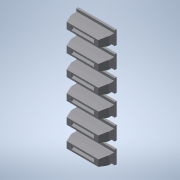
# Autodesk Inventor part: 0088-02-r2-coin-buttons-panelmot
Saved by Autodesk Inventor 2020.2 (Build 242310000, 310)
## iProperties
Created: 2011-08-20
Part Number: 0088-02-r2-coin-buttons-panelmot
Material: Allgemein
Document SubType Name: Modeling
Designer: Jaso
Density: 1 g/cm^3
Appearance: Vorgabe
Author: Jaso
Autodesk Inventor part; units mm, degrees
ref_plane "YZ Plane" through (0, 0, 0) normal (1, 0, 0) x (0, 1, 0)
ref_plane "XZ Plane" through (0, 0, 0) normal (0, 1, 0) x (-1, 0, 0)
sketch "Sketch1" plane through (0, 0, 0) normal (0, 0, 1) x (1, 0, 0)
  line L0 (-18.796, 63.5) -> (18.796, 63.5)
  line L1 (18.796, 63.5) -> (18.796, -63.5)
  line L2 (18.796, -63.5) -> (-18.796, -63.5)
  line L3 (-18.796, -63.5) -> (-18.796, 63.5)
  point P0 (0, 0)
  point P1 (18.796, 0)
  point P2 (0, 63.5)
  dimension "d0" = 127
  dimension "d1" = 37.592
  constraints: 8 end point, 2 midpoint, 2 parallel, 1 horizontal, 1 horizontal alignment, 1 perpendicular, 1 vertical alignment
  measures "d0" distance of L0.end L1.end
  measures "d1" distance between parallel lines of L3 L1
extrude "Extrusion1" add sketch "Sketch1" along normal blind 3.175
sketch "Sketch5" plane through (0, 0, 3.175) normal (0, 0, 1) x (1, 0, 0)
  line L0 (18.796, -63.5) -> (-18.796, -63.5) projected
  point P0 (0, 0)
  point P1 (0, -59.5376)
  point P2 (0, 59.5376)
  dimension "d22" = 119.0752
  dimension "d23" = 3.9624
  constraints: 2 vertical alignment
  measures "d22" distance of point (0, 59.538) point (0, -59.538)
  measures "d23" distance from line of point (0, -59.538) L0
hole "Hole1" at (0, -59.5376, 3.175) at (0, 59.5376, 3.175) direction (0, 0, -1) diameter 3.175 end through all
sketch "Sketch2" plane through (0, 0, 3.175) normal (0, 0, 1) x (1, 0, 0)
  line L0 (18.796, 63.5) -> (18.796, -63.5) projected
  line L1 (-18.796, -63.5) -> (-18.796, 63.5) projected
  line L2 (18.796, -63.5) -> (-18.796, -63.5) projected
  line L3 (-18.796, -45.8978) -> (18.796, -45.8978)
  line L4 (18.796, -45.8978) -> (18.796, -55.0418)
  line L5 (18.796, -55.0418) -> (-18.796, -55.0418)
  line L6 (-18.796, -55.0418) -> (-18.796, -45.8978)
  point P0 (0, 0)
  dimension "d4" = 9.144
  dimension "d5" = 8.4582
  constraints: 8 end point, 2 parallel, 2 point on line, 1 horizontal, 1 perpendicular
  measures "d4" distance between parallel lines of L3 L5
  measures "d5" distance between parallel lines of L5 L2
extrude "Extrusion2" add sketch "Sketch2" along normal blind 12.7 contours L0 L5 L1 L3
ref_plane "Work Plane1" through (0, 0, 24.8412) normal (0, 0, 1) x (1, 0, 0)
sketch "Sketch3" plane through (0, 0, 24.8412) normal (0, 0, 1) x (1, 0, 0)
  line L0 (18.796, -55.0418) -> (-18.796, -55.0418) projected
  line L1 (18.796, -45.8978) -> (18.796, -55.0418) projected
  line L2 (-18.796, -45.8978) -> (18.796, -45.8978) projected
  line L3 (-18.796, -55.0418) -> (-18.796, -45.8978) projected
  line L4 (-15.5321, -47.2948) -> (15.5321, -47.2948)
  line L5 (15.5321, -47.2948) -> (15.5321, -53.6448)
  line L6 (15.5321, -53.6448) -> (-15.5321, -53.6448)
  line L7 (-15.5321, -53.6448) -> (-15.5321, -47.2948)
  point P0 (0, 0)
  point P1 (15.5321, -50.4698)
  point P2 (18.796, -50.4698)
  point P3 (0, -45.8978)
  point P4 (0, -47.2948)
  dimension "d9" = 31.0642
  dimension "d10" = 6.35
  constraints: 8 end point, 4 midpoint, 2 parallel, 1 horizontal, 1 horizontal alignment, 1 perpendicular, 1 vertical alignment
  measures "d9" distance of L4.start L4.end
  measures "d10" distance of L4.end L5.end
loft "Loft1" add profiles "Sketch3" section 2 edges at (0, -55.0418, 15.875) (18.796, -50.4698, 15.875) (0, -45.8978, 15.875) (-18.796, -50.4698, 15.875) contours L4 L5 L6 L7
sketch "Sketch4" plane through (-15.5321, -47.2948, 24.8412) normal (0, 0, 1) x (1, 0, 0)
  line L0 (0, 0) -> (31.0642, 0) projected
  line L1 (31.0642, 0) -> (31.0642, -6.35) projected
  line L2 (4.4196, -1.5875) -> (26.6446, -1.5875)
  line L3 (26.6446, -1.5875) -> (26.6446, -4.7625)
  line L4 (26.6446, -4.7625) -> (4.4196, -4.7625)
  line L5 (4.4196, -4.7625) -> (4.4196, -1.5875)
  point P0 (15.5321, 47.2948)
  point P1 (26.6446, -3.175)
  point P2 (31.0642, -3.175)
  point P3 (15.5321, -1.5875)
  point P4 (15.5321, 0)
  dimension "d15" = 3.175
  dimension "d16" = 22.225
  constraints: 8 end point, 4 midpoint, 2 parallel, 1 horizontal, 1 horizontal alignment, 1 perpendicular, 1 vertical alignment
  measures "d15" distance of L2.end L3.end
  measures "d16" distance of L2.start L2.end
extrude "Extrusion3" cut sketch "Sketch4" against normal through all
pattern_linear "Rectangular Pattern1" count 6 spacing 20.193 along (0, 1, 0) of "Extrusion2", "Loft1", "Extrusion3"
sketch "Skizze6" plane through (0, 0, 3.175) normal (0, 0, 1) x (1, 0, 0)
  line L0 (-24.1756, 43.8912) -> (26.7048, 43.8912)
  line L1 (26.7048, 43.8912) -> (26.7048, 36.9062)
  line L2 (26.7048, 36.9062) -> (-24.1756, 36.9062)
  line L3 (-24.1756, 36.9062) -> (-24.1756, 43.8912)
  line L4 (-24.1756, 23.6982) -> (26.7048, 23.6982)
  line L5 (26.7048, 23.6982) -> (26.7048, 16.7132)
  line L6 (26.7048, 16.7132) -> (-24.1756, 16.7132)
  line L7 (-24.1756, 16.7132) -> (-24.1756, 23.6982)
  line L8 (-24.1756, 3.5052) -> (26.7048, 3.5052)
  line L9 (26.7048, 3.5052) -> (26.7048, -3.4798)
  line L10 (26.7048, -3.4798) -> (-24.1756, -3.4798)
  line L11 (-24.1756, -3.4798) -> (-24.1756, 3.5052)
  line L12 (-24.1756, -16.6878) -> (26.7048, -16.6878)
  line L13 (26.7048, -16.6878) -> (26.7048, -23.6728)
  line L14 (26.7048, -23.6728) -> (-24.1756, -23.6728)
  line L15 (-24.1756, -23.6728) -> (-24.1756, -16.6878)
  line L16 (-24.1756, 57.0992) -> (26.7048, 57.0992)
  line L17 (26.7048, 57.0992) -> (26.7048, 65.0866)
  line L18 (26.7048, 65.0866) -> (-24.1756, 65.0866)
  line L19 (-24.1756, 65.0866) -> (-24.1756, 57.0992)
  line L20 (-24.1756, -36.8808) -> (26.7048, -36.8808)
  line L21 (26.7048, -36.8808) -> (26.7048, -43.8658)
  line L22 (26.7048, -43.8658) -> (-24.1756, -43.8658)
  line L23 (-24.1756, -43.8658) -> (-24.1756, -36.8808)
  line L24 (-24.1756, -57.0738) -> (26.7048, -57.0738)
  line L25 (26.7048, -57.0738) -> (26.7048, -65.8307)
  line L26 (26.7048, -65.8307) -> (-24.1756, -65.8307)
  line L27 (-24.1756, -65.8307) -> (-24.1756, -57.0738)
  line L28 (-18.796, 55.0672) -> (18.796, 55.0672) projected
  line L29 (18.796, 45.9232) -> (-18.796, 45.9232) projected
  line L30 (-18.796, 34.8742) -> (18.796, 34.8742) projected
  line L31 (18.796, 25.7302) -> (-18.796, 25.7302) projected
  line L32 (-18.796, 14.6812) -> (18.796, 14.6812) projected
  line L33 (18.796, 5.5372) -> (-18.796, 5.5372) projected
  line L34 (-18.796, -5.5118) -> (18.796, -5.5118) projected
  line L35 (18.796, -14.6558) -> (-18.796, -14.6558) projected
  line L36 (-18.796, -25.7048) -> (18.796, -25.7048) projected
  line L37 (18.796, -34.8488) -> (-18.796, -34.8488) projected
  line L38 (-18.796, -45.8978) -> (18.796, -45.8978) projected
  line L39 (18.796, -55.0418) -> (-18.796, -55.0418) projected
  point P0 (0, 0)
  dimension "d31" = 2.032
  dimension "d32" = 2.032
  dimension "d33" = 2.032
  dimension "d34" = 2.032
  dimension "d35" = 2.032
  dimension "d36" = 2.032
  dimension "d37" = 2.032
  dimension "d38" = 2.032
  dimension "d39" = 2.032
  dimension "d40" = 2.032
  dimension "d41" = 2.032
  dimension "d42" = 2.032
  constraints: 56 end point, 14 parallel, 11 point on line, 7 horizontal, 7 perpendicular
  measures "d31" distance between parallel lines of L16 L28
  measures "d32" distance between parallel lines of L29 L0
  measures "d33" distance between parallel lines of L30 L2
  measures "d34" distance between parallel lines of L31 L4
  measures "d35" distance between parallel lines of L6 L32
  measures "d36" distance between parallel lines of L8 L33
  measures "d37" distance between parallel lines of L34 L10
  measures "d38" distance between parallel lines of L35 L12
  measures "d39" distance between parallel lines of L36 L14
  measures "d40" distance from line of L37 L20.end
  measures "d41" distance between parallel lines of L22 L38
  measures "d42" distance between parallel lines of L24 L39
extrude "Extrusion4" cut sketch "Skizze6" against normal blind 25.4
sketch "Skizze7" plane through (0, 0, 0) normal (0, 0, -1) x (-1, 0, 0)
  line L0 (18.796, 57.0992) -> (-18.796, 57.0992) projected
  line L1 (-18.796, 57.0992) -> (-18.796, 43.8912) projected
  line L2 (-18.796, 43.8912) -> (18.796, 43.8912) projected
  line L3 (18.796, 43.8912) -> (18.796, 57.0992) projected
  line L4 (-18.796, 55.0672) -> (-18.796, 45.9232) projected
  line L5 (-18.796, 50.4952) -> (18.796, 50.4952) construction
  line L6 (-11.1125, 48.9077) -> (-11.1125, 52.0827) projected
  circle A0 centre (-11.1125, 50.4952) radius 2
  line L7 (11.1125, 52.0827) -> (11.1125, 48.9077) projected
  circle A1 centre (11.1125, 50.4952) radius 2
  point P0 (0, 0)
  dimension "d45" = 4
  dimension "d46" = 4
  constraints: 4 midpoint, 2 centre point, 2 end point
  measures "d45" diameter of A0
  measures "d46" diameter of A1
extrude "Extrusion5" cut sketch "Skizze7" against normal blind 22.86 contours A0 | A1
sketch "Skizze8" plane through (0, 0, 0) normal (0, 0, -1) x (-1, 0, 0)
  line L0 (-1.9907, 52.4486) -> (2.0093, 52.4486)
  line L1 (2.0093, 52.4486) -> (2.0093, 48.4486)
  line L2 (2.0093, 48.4486) -> (-1.9907, 48.4486)
  line L3 (-1.9907, 48.4486) -> (-1.9907, 52.4486)
  line L4 (-1.9907, 52.4486) -> (2.0093, 48.4486) construction
  line L5 (2.0093, 52.4486) -> (-1.9907, 48.4486) construction
  point P0 (0, 0)
  point P1 (0.0093, 50.4486)
  dimension "d49" = 4
  dimension "d50" = 4
  constraints: 12 end point, 2 midpoint, 2 parallel, 1 horizontal, 1 perpendicular
  measures "d49" distance of L1.end L2.end
  measures "d50" distance of L0.end L1.end
extrude "Extrusion6" add sketch "Skizze8" against normal blind 5
sketch "Skizze10" plane through (0, 0, 0) normal (0, 0, -1) x (-1, 0, 0)
  line L0 (-19.2035, 30.2914) -> (18.796, 30.3022) construction
  line L1 (18.796, 23.6982) -> (18.796, 36.9062) projected
  line L2 (-19.1977, 9.8718) -> (18.796, 9.8718) construction
  line L3 (-18.796, -3.4798) -> (-18.796, -16.6878) projected
  line L4 (-18.796, -10.0838) -> (18.796, -10.0838) construction
  line L5 (-18.796, -23.6728) -> (-18.796, -36.8808) projected
  line L6 (-18.796, -30.2768) -> (18.796, -30.2768) construction
  line L7 (-18.796, -45.8978) -> (-18.796, -55.0418) projected
  line L8 (-18.796, -50.4698) -> (18.796, -50.4698) construction
  circle A0 centre (-11.0557, 30.2937) radius 2
  line L9 (11.1125, 31.8897) -> (11.1125, 28.7147) construction
  circle A1 centre (11.1125, 30.3022) radius 2
  line L10 (-11.1125, 8.5217) -> (-11.1125, 11.6967) construction
  circle A2 centre (-11.1125, 10.1092) radius 2
  line L11 (11.1125, 8.5217) -> (11.1125, 11.6967) construction
  circle A3 centre (11.1125, 10.1092) radius 2
  line L12 (-11.1125, -8.4963) -> (-11.1125, -11.6713) projected
  circle A4 centre (-11.1125, -10.0838) radius 2
  circle A5 centre (11.1125, -10.0838) radius 2
  line L13 (-11.1125, -31.8643) -> (-11.1125, -28.6893) projected
  circle A6 centre (-11.1125, -30.2768) radius 2
  line L14 (11.1125, -28.6893) -> (11.1125, -31.8643) projected
  circle A7 centre (11.1125, -30.2768) radius 2
  line L15 (-11.1125, -52.0573) -> (-11.1125, -48.8823) projected
  circle A8 centre (-11.1125, -50.4698) radius 2
  line L16 (11.1125, -48.8823) -> (11.1125, -52.0573) projected
  circle A9 centre (11.1125, -50.4698) radius 2
  point P0 (0, 0)
  dimension "d53" = 4
  dimension "d54" = 4
  dimension "d55" = 4
  dimension "d56" = 4
  dimension "d57" = 4
  dimension "d58" = 4
  dimension "d59" = 4
  dimension "d60" = 4
  dimension "d61" = 4
  dimension "d62" = 4
  constraints: 12 midpoint, 10 centre point, 10 end point, 4 horizontal, 2 point on line
  measures "d53" diameter of A0
  measures "d54" diameter of A1
  measures "d55" diameter of A2
  measures "d56" diameter of A3
  measures "d57" diameter of A4
  measures "d58" diameter of A5
  measures "d59" diameter of A6
  measures "d60" diameter of A7
  measures "d61" diameter of A8
  measures "d62" diameter of A9
extrude "Extrusion7" cut sketch "Skizze10" against normal blind 22.86
sketch "Skizze11" plane through (0, 0, 0) normal (0, 0, -1) x (-1, 0, 0)
  line L0 (-1.9772, 32.2984) -> (2.0228, 32.2984)
  line L1 (2.0228, 32.2984) -> (2.0228, 28.2984)
  line L2 (2.0228, 28.2984) -> (-1.9772, 28.2984)
  line L3 (-1.9772, 28.2984) -> (-1.9772, 32.2984)
  line L4 (-1.9772, 32.2984) -> (2.0228, 28.2984) construction
  line L5 (2.0228, 32.2984) -> (-1.9772, 28.2984) construction
  line L6 (-1.9661, 12.2651) -> (2.0339, 12.2651)
  line L7 (2.0339, 12.2651) -> (2.0339, 8.0041)
  line L8 (2.0339, 8.0041) -> (-1.9661, 8.0041)
  line L9 (-1.9661, 8.0041) -> (-1.9661, 12.2651)
  line L10 (-1.9661, 12.2651) -> (2.0339, 8.0041) construction
  line L11 (2.0339, 12.2651) -> (-1.9661, 8.0041) construction
  line L12 (-1.9772, -8.2024) -> (2.0228, -8.2024)
  line L13 (2.0228, -8.2024) -> (2.0228, -12.2024)
  line L14 (2.0228, -12.2024) -> (-1.9772, -12.2024)
  line L15 (-1.9772, -12.2024) -> (-1.9772, -8.2024)
  line L16 (-1.9772, -8.2024) -> (2.0228, -12.2024) construction
  line L17 (2.0228, -8.2024) -> (-1.9772, -12.2024) construction
  line L18 (-1.9772, -27.9157) -> (2.0228, -27.9157)
  line L19 (2.0228, -27.9157) -> (2.0228, -31.9157)
  line L20 (2.0228, -31.9157) -> (-1.9772, -31.9157)
  line L21 (-1.9772, -31.9157) -> (-1.9772, -27.9157)
  line L22 (-1.9772, -27.9157) -> (2.0228, -31.9157) construction
  line L23 (2.0228, -27.9157) -> (-1.9772, -31.9157) construction
  line L24 (-1.9772, -48.7043) -> (2.0228, -48.7043)
  line L25 (2.0228, -48.7043) -> (2.0228, -52.7043)
  line L26 (2.0228, -52.7043) -> (-1.9772, -52.7043)
  line L27 (-1.9772, -52.7043) -> (-1.9772, -48.7043)
  line L28 (-1.9772, -48.7043) -> (2.0228, -52.7043) construction
  line L29 (2.0228, -48.7043) -> (-1.9772, -52.7043) construction
  point P0 (0, 0)
  point P1 (0.0228, 30.2984)
  point P2 (0.0339, 10.1346)
  point P3 (0.0228, -10.2024)
  point P4 (0.0228, -29.9157)
  point P5 (0.0228, -50.7043)
  dimension "d65" = 4
  dimension "d66" = 4
  dimension "d67" = 4
  dimension "d68" = 4
  dimension "d69" = 4
  dimension "d70" = 4
  dimension "d71" = 4
  dimension "d72" = 4
  dimension "d73" = 4
  constraints: 60 end point, 10 midpoint, 10 parallel, 5 horizontal, 5 perpendicular
  measures "d65" distance of L1.end L2.end
  measures "d66" distance of L0.end L1.end
  measures "d67" distance of L7.end L8.end
  measures "d68" distance of L13.end L14.end
  measures "d69" distance of L12.end L13.end
  measures "d70" distance of L19.end L20.end
  measures "d71" distance of L18.end L19.end
  measures "d72" distance of L25.end L26.end
  measures "d73" distance of L24.end L25.end
extrude "Extrusion8" add sketch "Skizze11" against normal blind 5
sketch "Skizze12" plane through (-15.5321, 53.6702, 24.8412) normal (0, 0, 1) x (1, 0, 0)
  line L0 (-3.2639, 1.397) -> (34.3281, 1.397) projected
  line L1 (-3.2639, -7.747) -> (-3.2639, 1.397) projected
  line L2 (34.3281, -7.747) -> (-3.2639, -7.747) projected
  line L3 (34.3281, 1.397) -> (34.3281, -7.747) projected
  line L4 (-3.2639, -18.796) -> (34.3281, -18.796) projected
  line L5 (34.3281, -18.796) -> (34.3281, -27.94) projected
  line L6 (34.3281, -27.94) -> (-3.2639, -27.94) projected
  line L7 (-3.2639, -27.94) -> (-3.2639, -18.796) projected
  line L8 (-3.2639, -38.989) -> (34.3281, -38.989) projected
  line L9 (34.3281, -38.989) -> (34.3281, -48.133) projected
  line L10 (34.3281, -48.133) -> (-3.2639, -48.133) projected
  line L11 (-3.2639, -48.133) -> (-3.2639, -38.989) projected
  line L12 (-3.2639, -59.182) -> (34.3281, -59.182) projected
  line L13 (34.3281, -59.182) -> (34.3281, -68.326) projected
  line L14 (34.3281, -68.326) -> (-3.2639, -68.326) projected
  line L15 (-3.2639, -68.326) -> (-3.2639, -59.182) projected
  line L16 (-3.2639, -79.375) -> (34.3281, -79.375) projected
  line L17 (34.3281, -79.375) -> (34.3281, -88.519) projected
  line L18 (34.3281, -88.519) -> (-3.2639, -88.519) projected
  line L19 (-3.2639, -88.519) -> (-3.2639, -79.375) projected
  line L20 (-3.2639, -99.568) -> (34.3281, -99.568) projected
  line L21 (-3.2639, -108.712) -> (-3.2639, -99.568) projected
  line L22 (34.3281, -108.712) -> (-3.2639, -108.712) projected
  line L23 (34.3281, -99.568) -> (34.3281, -108.712) projected
  line L24 (33.8281, 0.897) -> (-2.7639, 0.897)
  line L25 (-2.7639, 0.897) -> (-2.7639, -7.247)
  line L26 (-2.7639, -7.247) -> (33.8281, -7.247)
  line L27 (33.8281, -7.247) -> (33.8281, 0.897)
  line L28 (33.8281, -19.296) -> (-2.7639, -19.296)
  line L29 (-2.7639, -19.296) -> (-2.7639, -27.44)
  line L30 (-2.7639, -27.44) -> (33.8281, -27.44)
  line L31 (33.8281, -27.44) -> (33.8281, -19.296)
  line L32 (33.8281, -39.489) -> (-2.7639, -39.489)
  line L33 (-2.7639, -39.489) -> (-2.7639, -47.633)
  line L34 (-2.7639, -47.633) -> (33.8281, -47.633)
  line L35 (33.8281, -47.633) -> (33.8281, -39.489)
  line L36 (33.8281, -59.682) -> (-2.7639, -59.682)
  line L37 (-2.7639, -59.682) -> (-2.7639, -67.826)
  line L38 (-2.7639, -67.826) -> (33.8281, -67.826)
  line L39 (33.8281, -67.826) -> (33.8281, -59.682)
  line L40 (33.8281, -79.875) -> (-2.7639, -79.875)
  line L41 (-2.7639, -79.875) -> (-2.7639, -88.019)
  line L42 (-2.7639, -88.019) -> (33.8281, -88.019)
  line L43 (33.8281, -88.019) -> (33.8281, -79.875)
  line L44 (33.8281, -100.068) -> (-2.7639, -100.068)
  line L45 (-2.7639, -100.068) -> (-2.7639, -108.212)
  line L46 (-2.7639, -108.212) -> (33.8281, -108.212)
  line L47 (33.8281, -108.212) -> (33.8281, -100.068)
  point P0 (15.5321, -53.6702)
  dimension "d76" = 0.5
  dimension "d77" = 0.5
  dimension "d78" = 0.5
  dimension "d79" = 0.5
  dimension "d80" = 0.5
  dimension "d81" = 0.5
  constraints: 48 end point, 18 other
  measures "d76" distance between parallel lines of L0 L24
  measures "d77" distance between parallel lines of L4 L28
  measures "d78" distance between parallel lines of L8 L32
  measures "d79" distance between parallel lines of L12 L36
  measures "d80" distance between parallel lines of L16 L40
  measures "d81" distance between parallel lines of L20 L44
extrude "Extrusion9" cut sketch "Skizze12" against normal up to surface (21.6662 mm away)
sketch "Bottom" plane through (0, 0, 0) normal (0, 0, -1) x (-1, 0, 0)
  line L0 (-1.9907, 48.9077) -> (-9.896, 48.9077) projected
  arc A0 (-9.896, 52.0827) -> (-9.896, 48.9077) centre (-11.1125, 50.4952) ccw projected
  line L1 (-9.896, 52.0827) -> (-1.9907, 52.0827) projected
  line L2 (-1.9907, 48.9077) -> (-1.9907, 52.0827) projected
  line L3 (2.0093, 52.0827) -> (2.0093, 48.9077) projected
  line L4 (2.0093, 52.0827) -> (9.896, 52.0827) projected
  arc A1 (9.896, 48.9077) -> (9.896, 52.0827) centre (11.1125, 50.4952) ccw projected
  line L5 (9.896, 48.9077) -> (2.0093, 48.9077) projected
  line L6 (18.796, 57.0992) -> (-18.796, 57.0992) projected
  line L7 (-18.796, 57.0992) -> (-18.796, 43.8912) projected
  line L8 (-18.796, 43.8912) -> (18.796, 43.8912) projected
  line L9 (18.796, 43.8912) -> (18.796, 57.0992) projected
  line L10 (-1.9772, 28.7147) -> (-9.8283, 28.7147) projected
  arc A2 (-9.8504, 31.8897) -> (-9.8283, 28.7147) centre (-11.0557, 30.2937) ccw projected
  line L11 (-9.8504, 31.8897) -> (-1.9772, 31.8897) projected
  line L12 (-1.9772, 28.7147) -> (-1.9772, 31.8897) projected
  line L13 (2.0228, 31.8897) -> (2.0228, 28.7147) projected
  line L14 (2.0228, 31.8897) -> (9.896, 31.8897) projected
  arc A3 (9.896, 28.7147) -> (9.896, 31.8897) centre (11.1125, 30.3022) ccw projected
  line L15 (9.896, 28.7147) -> (2.0228, 28.7147) projected
  line L16 (-18.796, 23.6982) -> (18.796, 23.6982) projected
  line L17 (18.796, 23.6982) -> (18.796, 36.9062) projected
  line L18 (18.796, 36.9062) -> (-18.796, 36.9062) projected
  line L19 (-18.796, 36.9062) -> (-18.796, 23.6982) projected
  line L20 (-1.9661, 8.5217) -> (-9.896, 8.5217) projected
  arc A4 (-9.896, 11.6967) -> (-9.896, 8.5217) centre (-11.1125, 10.1092) ccw projected
  line L21 (-9.896, 11.6967) -> (-1.9661, 11.6967) projected
  line L22 (-1.9661, 8.5217) -> (-1.9661, 11.6967) projected
  line L23 (2.0339, 11.6967) -> (2.0339, 8.5217) projected
  line L24 (2.0339, 11.6967) -> (9.896, 11.6967) projected
  arc A5 (9.896, 8.5217) -> (9.896, 11.6967) centre (11.1125, 10.1092) ccw projected
  line L25 (9.896, 8.5217) -> (2.0339, 8.5217) projected
  line L26 (18.796, 16.7132) -> (-18.796, 16.7132) projected
  line L27 (-18.796, 16.7132) -> (-18.796, 3.5052) projected
  line L28 (-18.796, 3.5052) -> (18.796, 3.5052) projected
  line L29 (18.796, 3.5052) -> (18.796, 16.7132) projected
  line L30 (-1.9772, -11.6713) -> (-9.896, -11.6713) projected
  arc A6 (-9.896, -8.4963) -> (-9.896, -11.6713) centre (-11.1125, -10.0838) ccw projected
  line L31 (-9.896, -8.4963) -> (-1.9772, -8.4963) projected
  line L32 (-1.9772, -11.6713) -> (-1.9772, -8.4963) projected
  line L33 (2.0228, -8.4963) -> (2.0228, -11.6713) projected
  line L34 (2.0228, -8.4963) -> (9.896, -8.4963) projected
  arc A7 (9.896, -11.6713) -> (9.896, -8.4963) centre (11.1125, -10.0838) ccw projected
  line L35 (9.896, -11.6713) -> (2.0228, -11.6713) projected
  line L36 (-18.796, -16.6878) -> (18.796, -16.6878) projected
  line L37 (18.796, -16.6878) -> (18.796, -3.4798) projected
  line L38 (18.796, -3.4798) -> (-18.796, -3.4798) projected
  line L39 (-18.796, -3.4798) -> (-18.796, -16.6878) projected
  line L40 (-1.9772, -31.8643) -> (-9.896, -31.8643) projected
  arc A8 (-9.896, -28.6893) -> (-9.896, -31.8643) centre (-11.1125, -30.2768) ccw projected
  line L41 (-9.896, -28.6893) -> (-1.9772, -28.6893) projected
  line L42 (-1.9772, -31.8643) -> (-1.9772, -28.6893) projected
  line L43 (2.0228, -28.6893) -> (2.0228, -31.8643) projected
  line L44 (2.0228, -28.6893) -> (9.896, -28.6893) projected
  arc A9 (9.896, -31.8643) -> (9.896, -28.6893) centre (11.1125, -30.2768) ccw projected
  line L45 (9.896, -31.8643) -> (2.0228, -31.8643) projected
  line L46 (18.796, -23.6728) -> (-18.796, -23.6728) projected
  line L47 (-18.796, -23.6728) -> (-18.796, -36.8808) projected
  line L48 (-18.796, -36.8808) -> (18.796, -36.8808) projected
  line L49 (18.796, -36.8808) -> (18.796, -23.6728) projected
  line L50 (-1.9772, -52.0573) -> (-9.896, -52.0573) projected
  arc A10 (-9.896, -48.8823) -> (-9.896, -52.0573) centre (-11.1125, -50.4698) ccw projected
  line L51 (-9.896, -48.8823) -> (-1.9772, -48.8823) projected
  line L52 (-1.9772, -52.0573) -> (-1.9772, -48.8823) projected
  line L53 (2.0228, -48.8823) -> (2.0228, -52.0573) projected
  line L54 (2.0228, -48.8823) -> (9.896, -48.8823) projected
  arc A11 (9.896, -52.0573) -> (9.896, -48.8823) centre (11.1125, -50.4698) ccw projected
  line L55 (9.896, -52.0573) -> (2.0228, -52.0573) projected
  line L56 (18.796, -43.8658) -> (-18.796, -43.8658) projected
  line L57 (-18.796, -43.8658) -> (-18.796, -57.0738) projected
  line L58 (-18.796, -57.0738) -> (18.796, -57.0738) projected
  line L59 (18.796, -57.0738) -> (18.796, -43.8658) projected
  point P0 (0, 0)
sketch "Skizze14" plane through (-18.796, 57.0992, 3.175) normal (0, 1, 0) x (1, 0, 0)
  line L0 (-4.3658, -9) -> (41.2147, -9)
  line L1 (41.2147, -9) -> (41.2147, 7.4573)
  line L2 (41.2147, 7.4573) -> (-4.3658, 7.4573)
  line L3 (-4.3658, 7.4573) -> (-4.3658, -9)
  point P0 (18.796, 3.175)
  point P1 (0, 0)
  dimension "d84" = 9
  constraints: 8 end point, 2 parallel, 1 horizontal, 1 perpendicular
  measures "d84" distance from line of L0 point (0, 0)
extrude "Extrusion10" cut sketch "Skizze14" against normal through all
sketch "Skizze15" plane through (18.296, 46.4232, 12.175) normal (0, 0, -1) x (-1, 0, 0)
  point P0 (18.296, -46.4232)
extrude "Extrusion11" add sketch "Bottom" against normal blind 12.175
sketch "Skizze16" plane through (-18.796, 57.0992, 0) normal (0, 1, 0) x (1, 0, 0)
  line L0 (0, 0) -> (37.592, 0) projected
  line L1 (0, 0) -> (0, -12.175) projected
  line L2 (37.592, -12.175) -> (0, -12.175) projected
  line L3 (37.592, 0) -> (37.592, -12.175) projected
  line L4 (-4.7241, 4.5643) -> (43.4575, 4.5643)
  line L5 (43.4575, 4.5643) -> (43.4575, -10.175)
  line L6 (43.4575, -10.175) -> (-4.7241, -10.175)
  line L7 (-4.7241, -10.175) -> (-4.7241, 4.5643)
  point P0 (18.796, 0)
  dimension "d89" = 2
  constraints: 8 end point, 2 parallel, 1 horizontal, 1 perpendicular
  measures "d89" distance between parallel lines of L6 L2
extrude "Extrusion12" cut sketch "Skizze16" against normal through all contours L1 L6 L7 L4 L5 L3 L0 | L0 L3 L6 L1
body "Solid1"
